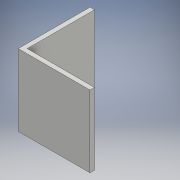
# Autodesk Inventor part: Lframe_corner
Saved by Autodesk Inventor 2018 (Build 220112000, 112)
## iProperties
Created: 2018-10-27
Part Number: Lframe_corner
Material: Generic
Document SubType Name: Modeling
Designer: Fredy Espana C
Density: 1 g/cm^3
Appearance: Default
Author: Fredy Espana C
Autodesk Inventor part; units mm, degrees
ref_plane "YZ Plane" through (0, 0, 0) normal (1, 0, 0) x (0, 1, 0)
ref_plane "XZ Plane" through (0, 0, 0) normal (0, 1, 0) x (-1, 0, 0)
ref_plane "XY Plane" through (0, 0, 0) normal (0, 0, 1) x (1, 0, 0)
sketch "Sketch1" plane through (0, 0, 0) normal (0, 0, 1) x (1, 0, 0)
  line L0 (0, 0) -> (3.7711, 0)
  line L1 (1.5875, 1.5875) -> (1.5875, 25.4)
  line L2 (1.5875, 25.4) -> (0, 25.4)
  line L3 (0, 25.4) -> (0, 0)
  line L4 (1.5875, 1.5875) -> (25.4, 1.5875)
  line L5 (25.4, 1.5875) -> (25.4, 0)
  line L6 (25.4, 0) -> (0, 0)
  line L7 (0, 0) -> (0, 4.2577)
  dimension "d0" = 25.4
  dimension "d1" = 25.4
  dimension "d2" = 1.5875
  dimension "d3" = 1.5875
  constraints: 16 end point, 4 parallel, 2 horizontal, 2 perpendicular, 2 point on line
  measures "d0" distance of L2.end L0.start
  measures "d1" distance of L5.end L6.end
  measures "d2" distance of L4.end L5.end
  measures "d3" distance of L1.end L2.end
extrude "Extrusion1" add sketch "Sketch1" along normal blind 25.4
body "Solid1"
